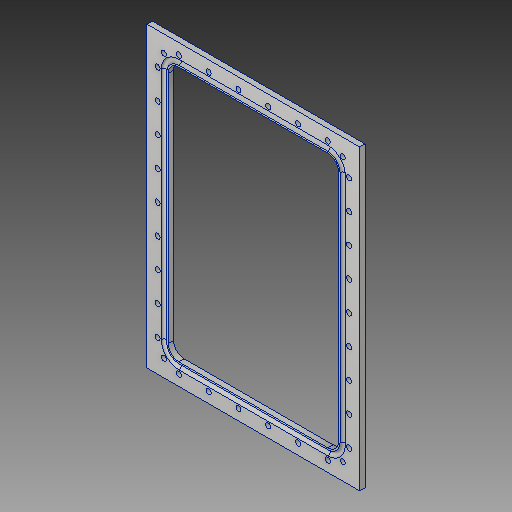
# Autodesk Inventor part: alumbottom3
Saved by Autodesk Inventor 2018.1 (Build 221171000, 171)
## iProperties
Created: 2017-08-02
Part Number: alumbottom3
Material: Aluminum 6061
Document SubType Name: Modeling
Designer: Kai
Density: 2.7 g/cm^3
Appearance: Aluminum - Flat
Author: Kai
Autodesk Inventor part; units mm, degrees
ref_plane "YZ Plane" through (0, 0, 0) normal (1, 0, 0) x (0, 1, 0)
ref_plane "XZ Plane" through (0, 0, 0) normal (0, 1, 0) x (-1, 0, 0)
sketch "Sketch1" plane through (0, 0, 0) normal (0, 0, 1) x (1, 0, 0)
  line L0 (0, 0) -> (254, 0)
  line L1 (254, 0) -> (254, 355.6)
  line L2 (254, 355.6) -> (0, 355.6)
  line L3 (0, 355.6) -> (0, 0)
  dimension "d0" = 254
  dimension "d1" = 355.6
  constraints: 8 end point, 2 parallel, 1 horizontal, 1 perpendicular
  measures "d0" distance of L2.end L1.end
  measures "d1" distance of L1.end L0.end
extrude "Extrusion1" add sketch "Sketch1" along normal blind 6.35
sketch "Sketch2" plane through (0, 0, 6.35) normal (0, 0, 1) x (1, 0, 0)
  line L0 (38.1, 342.9) -> (215.9, 342.9) construction
  line L1 (241.3, 317.5) -> (241.3, 38.1) construction
  line L2 (215.9, 12.7) -> (38.1, 12.7) construction
  line L3 (12.7, 38.1) -> (12.7, 317.5) construction
  line L4 (0, 355.6) -> (0, 0) construction
  line L5 (254, 355.6) -> (0, 355.6) construction
  arc A0 (241.3, 317.5) -> (215.9, 342.9) centre (215.9, 317.5) ccw construction
  arc A1 (38.1, 342.9) -> (12.7, 317.5) centre (38.1, 317.5) ccw construction
  arc A2 (12.7, 38.1) -> (38.1, 12.7) centre (38.1, 38.1) ccw construction
  arc A3 (215.9, 12.7) -> (241.3, 38.1) centre (215.9, 38.1) ccw construction
  line L6 (215.9, 38.1) -> (233.8605, 20.1395) construction
  line L7 (38.1, 38.1) -> (20.1395, 20.1395) construction
  line L8 (38.1, 317.5) -> (20.1395, 335.4605) construction
  line L9 (215.9, 317.5) -> (233.8605, 335.4605) construction
  circle A4 centre (20.1395, 335.4605) radius 3.1
  circle A5 centre (233.8605, 335.4605) radius 3.1
  circle A6 centre (233.8605, 20.1395) radius 3.1
  circle A7 centre (20.1395, 20.1395) radius 3.1
  circle A8 centre (12.7, 38.1) radius 3.1
  circle A9 centre (38.1, 12.7) radius 3.1
  circle A10 centre (215.9, 12.7) radius 3.1
  circle A11 centre (241.3, 38.1) radius 3.1
  circle A12 centre (241.3, 317.5) radius 3.1
  circle A13 centre (215.9, 342.9) radius 3.1
  circle A14 centre (38.1, 342.9) radius 3.1
  circle A15 centre (12.7, 317.5) radius 3.1
  circle A16 centre (241.3, 282.575) radius 3.1
  circle A17 centre (241.3, 247.65) radius 3.1
  circle A18 centre (241.3, 212.725) radius 3.1
  circle A19 centre (241.3, 177.8) radius 3.1
  circle A20 centre (241.3, 142.875) radius 3.1
  circle A21 centre (180.34, 342.9) radius 3.1
  circle A22 centre (144.78, 342.9) radius 3.1
  circle A23 centre (109.22, 342.9) radius 3.1
  circle A24 centre (73.66, 342.9) radius 3.1
  circle A25 centre (180.34, 12.7) radius 3.1
  circle A26 centre (144.78, 12.7) radius 3.1
  circle A27 centre (109.22, 12.7) radius 3.1
  circle A28 centre (73.66, 12.7) radius 3.1
  circle A29 centre (241.3, 107.95) radius 3.1
  circle A30 centre (241.3, 73.025) radius 3.1
  circle A31 centre (241.3, 38.1) radius 3.1
  circle A32 centre (12.7, 282.575) radius 3.1
  circle A33 centre (12.7, 247.65) radius 3.1
  circle A34 centre (12.7, 212.725) radius 3.1
  circle A35 centre (12.7, 177.8) radius 3.1
  circle A36 centre (12.7, 142.875) radius 3.1
  circle A37 centre (12.7, 107.95) radius 3.1
  circle A38 centre (12.7, 73.025) radius 3.1
  point P0 (241.3, 12.7)
  point P1 (241.3, 342.9)
  point P2 (12.7, 12.7)
  dimension "d4" = 228.6
  dimension "d5" = 330.2
  dimension "d6" = 12.7
  dimension "d7" = 12.7
  dimension "d8" = 25.4
  dimension "d9" = 6.2
  dimension "d10" = 6.2
  dimension "d11" = 6.2
  dimension "d12" = 6.2
  dimension "d13" = 6.2
  dimension "d14" = 6.2
  dimension "d15" = 6.2
  dimension "d16" = 6.2
  dimension "d17" = 6.2
  dimension "d18" = 6.2
  dimension "d19" = 6.2
  dimension "d20" = 6.2
  dimension "d30" = 34.925
  dimension "d37" = 35.56
  dimension "d44" = 35.56
  dimension "d51" = 0
  dimension "d52" = 0
  dimension "d53" = 0
  dimension "d54" = 0
  dimension "d57" = 34.925
  constraints: 39 centre point, 16 end point, 12 point on circle, 8 tangent, 6 point on line, 5 coincident, 3 equal radius, 3 horizontal, 2 parallel, 2 vertical, 1 perpendicular, 46 other
  measures "d4" distance of point (241.3, 12.7) point (12.7, 12.7)
  measures "d5" distance of point (241.3, 342.9) point (241.3, 12.7)
  measures "d6" distance between parallel lines of L4 L3
  measures "d7" distance between parallel lines of L5 L0
  measures "d8" radius of A0
  measures "d9" diameter of A4
  measures "d10" diameter of A5
  measures "d11" diameter of A6
  measures "d12" diameter of A7
  measures "d13" diameter of A8
  measures "d14" diameter of A9
  measures "d15" diameter of A10
  measures "d16" diameter of A11
  measures "d17" diameter of A12
  measures "d18" diameter of A13
  measures "d19" diameter of A14
  measures "d20" diameter of A15
  measures "d30" distance of A12.centre A16.centre
  measures "d37" distance of A13.centre A21.centre
  measures "d44" distance of A10.centre A25.centre
  measures "d51" distance from line of L0 A14.centre
  measures "d52" distance from line of L0 A13.centre
  measures "d53" distance of L3.end A15.centre
  measures "d54" distance of L1.start A12.centre
  measures "d57" distance of A15.centre A32.centre
extrude "Extrusion2" cut sketch "Sketch2" against normal blind 12.7
sketch "Sketch3" plane through (0, 0, 6.35) normal (0, 0, 1) x (1, 0, 0)
  line L0 (38.1, 335.28) -> (215.9, 335.28)
  line L1 (233.68, 317.5) -> (233.68, 38.1)
  line L2 (215.9, 20.32) -> (38.1, 20.32)
  line L3 (20.32, 38.1) -> (20.32, 317.5)
  line L4 (254, 355.6) -> (0, 355.6) projected
  line L5 (0, 355.6) -> (0, 0) projected
  arc A0 (38.1, 335.28) -> (20.32, 317.5) centre (38.1, 317.5) ccw
  arc A1 (233.68, 317.5) -> (215.9, 335.28) centre (215.9, 317.5) ccw
  arc A2 (215.9, 20.32) -> (233.68, 38.1) centre (215.9, 38.1) ccw
  arc A3 (20.32, 38.1) -> (38.1, 20.32) centre (38.1, 38.1) ccw
  point P0 (233.68, 20.32)
  point P1 (233.68, 335.28)
  point P2 (20.32, 20.32)
  dimension "d62" = 213.36
  dimension "d63" = 314.96
  dimension "d64" = 20.32
  dimension "d65" = 20.32
  dimension "d66" = 17.78
  constraints: 8 end point, 8 point on circle, 8 tangent, 6 point on line, 4 centre point, 3 equal radius, 2 parallel, 1 horizontal, 1 perpendicular
  measures "d62" distance of point (233.68, 20.32) point (20.32, 20.32)
  measures "d63" distance of point (233.68, 335.28) point (233.68, 20.32)
  measures "d64" distance between parallel lines of L4 L0
  measures "d65" distance between parallel lines of L5 L3
  measures "d66" radius of A0
ref_plane "Work Plane1" through (0, 304.8, 0) normal (0, 1, 0) x (1, 0, 0)
sketch "Sketch5" plane through (0, 304.8, 0) normal (0, 1, 0) x (1, 0, 0)
  line L0 (0, -6.35) -> (254, -6.35) projected
  circle A0 centre (20.32, -6.35) radius 3.175
  line L1 (0, 0) -> (0, -6.35) projected
  dimension "d70" = 6.35
  dimension "d71" = 20.32
  constraints: 1 centre point, 1 point on line
  measures "d70" diameter of A0
  measures "d71" distance from line of L1 A0.centre
sweep "Sweep1" cut profiles "Sketch5" path "Sketch3" path curves L3 A3 L2 A2 L1 A1 L0 A0
sketch "Sketch6" plane through (0, 0, 6.35) normal (0, 0, 1) x (1, 0, 0)
  line L0 (38.1, 330.2) -> (215.9, 330.2)
  line L1 (228.6, 317.5) -> (228.6, 38.1)
  line L2 (215.9, 25.4) -> (38.1, 25.4)
  line L3 (25.4, 38.1) -> (25.4, 317.5)
  line L4 (0, 355.6) -> (0, 0) projected
  line L5 (254, 355.6) -> (0, 355.6) projected
  arc A0 (38.1, 330.2) -> (25.4, 317.5) centre (38.1, 317.5) ccw
  arc A1 (228.6, 317.5) -> (215.9, 330.2) centre (215.9, 317.5) ccw
  arc A2 (215.9, 25.4) -> (228.6, 38.1) centre (215.9, 38.1) ccw
  arc A3 (25.4, 38.1) -> (38.1, 25.4) centre (38.1, 38.1) ccw
  point P0 (228.6, 25.4)
  point P1 (228.6, 330.2)
  point P2 (25.4, 25.4)
  dimension "d74" = 203.2
  dimension "d75" = 304.8
  dimension "d76" = 25.4
  dimension "d77" = 25.4
  dimension "d78" = 12.7
  constraints: 8 end point, 8 point on circle, 8 tangent, 6 point on line, 4 centre point, 3 equal radius, 2 parallel, 1 horizontal, 1 perpendicular
  measures "d74" distance of point (228.6, 25.4) point (25.4, 25.4)
  measures "d75" distance of point (228.6, 330.2) point (228.6, 25.4)
  measures "d76" distance between parallel lines of L4 L3
  measures "d77" distance between parallel lines of L5 L0
  measures "d78" radius of A0
extrude "Extrusion3" cut sketch "Sketch6" against normal blind 25.4
body "Solid1"
